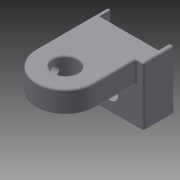
# Autodesk Inventor part: 6mmRingBracketRight
Saved by Autodesk Inventor 2014 SP1 (Build 180222100, 222)
## iProperties
Created: 2016-11-27
Part Number: 6mmRingBracketRight
Material: Generic
Document SubType Name: Modeling
Designer: danielsikar
Density: 1 g/cm^3
Appearance: Default
Author: danielsikar
Autodesk Inventor part; units mm, degrees
ref_plane "YZ Plane" through (0, 0, 0) normal (1, 0, 0) x (0, 1, 0)
ref_plane "XZ Plane" through (0, 0, 0) normal (0, 1, 0) x (-1, 0, 0)
ref_plane "XY Plane" through (0, 0, 0) normal (0, 0, 1) x (1, 0, 0)
sketch "Sketch1" plane through (0, 0, 0) normal (0, 0, 1) x (1, 0, 0)
  circle A0 centre (0, 0) radius 3.25
  circle A1 centre (0, 0) radius 8
  dimension "d0" = 6.5
  dimension "d1" = 16
  constraints: 2 centre point, 2 coincident
  measures "d0" diameter of A0
  measures "d1" diameter of A1
extrude "Extrusion1" add sketch "Sketch1" along normal blind 6
sketch "Sketch2" plane through (0, 0, 0) normal (1, 0, 0) x (0, 1, 0)
  circle A0 centre (0, 3) radius 1.25
  line L0 (-8, 0) -> (8, 0) projected
  point P0 (0, 0)
  dimension "d4" = 2.5
  dimension "d39" = 3
  constraints: 1 centre point
  measures "d4" diameter of A0
  measures "d39" distance from line of L0 A0.centre
extrude "Extrusion2" cut sketch "Sketch2" against normal blind 20
fillet "Fillet1" radius 0.5 1 edges at (-8, 0, 6)
fillet "Fillet2" radius 0.5 4 edges at (-7.9017, -1.25, 2.9978) (-8, 0, 0) (-3.25, 0, 0) (-3.25, 0, 6)
sketch "Sketch3" plane through (0, 0, 6) normal (0, 0, 1) x (1, 0, 0)
  circle A0 centre (0, 0) radius 7.5 projected
  line L0 (-8, 0) -> (8, 0)
  line L1 (8, 0) -> (8, 19)
  line L2 (8, 19) -> (-8, 19)
  line L3 (-8, 19) -> (-8, 0)
  dimension "d9" = 16
  dimension "d10" = 19
  dimension "d11" = 8
  dimension "d17" = 0
  constraints: 8 end point, 2 parallel, 1 horizontal, 1 perpendicular
  measures "d9" distance of L2.end L1.end
  measures "d10" distance of L1.end L0.end
  measures "d11" distance from line of A0.centre L3
  measures "d17" distance from line of A0.centre L0
extrude "Extrusion3" add sketch "Sketch3" against normal blind 6 contours L0 A0 | A0 L0 L3 L2 L1 picked at (-1.3085, 5.1375)
sketch "Sketch4" plane through (0, 0, 0) normal (0, 0, -1) x (-1, 0, 0)
  line L0 (8, 0) -> (8, 19) projected
  line L1 (-8, 19) -> (8, 19)
  line L2 (8, 19) -> (8, 11)
  line L3 (8, 11) -> (-8, 11)
  line L4 (-8, 11) -> (-8, 19)
  dimension "d14" = 8
  constraints: 8 end point, 2 parallel, 1 horizontal, 1 perpendicular, 1 point on line
  measures "d14" distance of L1.end L2.end
extrude "Extrusion4" add sketch "Sketch4" along normal blind 10
sketch "Sketch5" plane through (-8, 19, 6) normal (0, 1, 0) x (1, 0, 0)
  line L0 (16, 0) -> (16, 16) projected
  line L1 (0, 16) -> (16, 16) projected
  circle A0 centre (8.9, 11) radius 2.2
  point P0 (8, 6)
  dimension "d18" = 4.4
  dimension "d19" = 7.1
  dimension "d20" = 5
  constraints: 1 centre point
  measures "d18" diameter of A0
  measures "d19" distance from line of L0 A0.centre
  measures "d20" distance from line of A0.centre L1
extrude "Extrusion5" cut sketch "Sketch5" against normal blind 10
sketch "Sketch6" plane through (8, 0, 6) normal (1, 0, 0) x (0, 0, -1)
  line L0 (16, 19) -> (16, 11) projected
  line L1 (0, 19) -> (16, 19) projected
  line L2 (0, 19) -> (16, 19)
  line L3 (16, 19) -> (16, 11)
  line L4 (16, 11) -> (0, 11)
  line L5 (0, 11) -> (0, 19)
  constraints: 8 end point, 2 parallel, 1 horizontal, 1 perpendicular
extrude "Extrusion6" add sketch "Sketch6" along normal blind 2
sketch "Sketch7" plane through (-8, 19, 6) normal (0, 1, 0) x (1, 0, 0)
  circle A0 centre (8.9, 11) radius 2.2 projected
  line L0 (18, 0) -> (0, 0) projected
  line L1 (18, 16) -> (18, 0) projected
  line L2 (0, 16) -> (18, 16) projected
  line L3 (17, 0) -> (1, 0)
  line L4 (1, 0) -> (1, 16)
  line L5 (1, 16) -> (17, 16)
  line L6 (17, 16) -> (17, 0)
  point P0 (8, 6)
  dimension "d25" = 16
  dimension "d26" = 1
  constraints: 8 end point, 2 parallel, 2 point on line, 1 horizontal, 1 perpendicular
  measures "d25" distance of L4.end L5.end
  measures "d26" distance between parallel lines of L1 L6
extrude "Extrusion7" cut sketch "Sketch7" against normal blind 3 contours L0 L4 L2 L6
sketch "Sketch8" plane through (0, 0, 0) normal (0, 0, -1) x (-1, 0, 0)
  arc A0 (-3.75, 0) -> (3.75, 0) centre (0, 0) ccw projected
  circle A1 centre (0, 0) radius 3.25
  dimension "d29" = 6.5
  constraints: 1 centre point, 1 coincident
  measures "d29" diameter of A1
extrude "Extrusion8" cut sketch "Sketch8" against normal through all
fillet "Fillet3" radius 0.5 1 edges at (0, 3.25, 0)
fillet "Fillet4" radius 0.5 1 edges at (0, 3.25, 6)
fillet "Fillet5" radius 0.5 13 edges at (-8, 9.5, 6) (-8, 5.5, 0) (-8, 11, -5) (-8, 15, -10) (1, 11, -10) (-8, 19, -2) (10, 11, -2) (8, 5.5, 0) (8, 11, 3) (8, 5.5, 6) (10, 15, 6) (9, 11, 6) (10, 15, -10)
sketch "Sketch9" plane through (-8, 0, 1.25) normal (-1, 0, 0) x (0, 0, 1)
  line L0 (3.5, 0) -> (0, 0) projected
  circle A0 centre (1.75, 0) radius 1.25
  point P0 (-1.25, 0)
  dimension "d35" = 2.5
  constraints: 1 centre point, 1 midpoint
  measures "d35" diameter of A0
extrude "Extrusion9" cut sketch "Sketch9" against normal blind 8
fillet "Fillet6" radius 0.5 1 edges at (-8, 1.25, 3)
body "Solid1"
